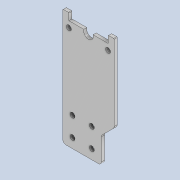
# Autodesk Inventor part: X Axis Statonary Composite Belt Holder RIGHT
Saved by Autodesk Inventor 2022 (Build 260153000, 153)
## iProperties
Created: 2021-10-21
Part Number: X Axis Statonary Composite Belt Holder RIGHT
Material: Generic
Document SubType Name: Modeling
Designer: Coy
Density: 1 g/cm^3
Appearance: Machined - Aluminum
Author: Coy
Autodesk Inventor part; units mm, degrees
ref_plane "YZ Plane" through (0, 0, 0) normal (1, 0, 0) x (0, 1, 0)
ref_plane "XZ Plane" through (0, 0, 0) normal (0, 1, 0) x (-1, 0, 0)
ref_plane "XY Plane" through (0, 0, 0) normal (0, 0, 1) x (1, 0, 0)
sketch "Sketch1" plane through (0, 0, 0) normal (0, 0, 1) x (1, 0, 0)
  line L0 (0, 0) -> (-40, 0)
  line L1 (-40, 0) -> (-40, 40)
  line L2 (-40, 40) -> (0, 40)
  line L3 (0, 40) -> (0, 0)
  line L4 (-30, 30) -> (-10, 30) construction
  line L5 (-10, 30) -> (-10, 10) construction
  line L6 (-10, 10) -> (-30, 10) construction
  line L7 (-30, 10) -> (-30, 30) construction
  line L8 (-30, 30) -> (-40, 30) construction
  line L9 (-10, 10) -> (0, 10) construction
  circle A0 centre (-30, 30) radius 2.6
  circle A1 centre (-10, 30) radius 2.6
  circle A2 centre (-10, 10) radius 2.6
  circle A3 centre (-30, 10) radius 2.6
  line L10 (-40, 40) -> (13, 40)
  line L11 (13, 40) -> (13, 100)
  line L12 (13, 100) -> (-40, 100)
  line L13 (-40, 100) -> (-40, 40)
  line L14 (13, 40) -> (0, 27)
  line L15 (-40, 100) -> (13, 100)
  line L16 (13, 100) -> (13, 120)
  line L17 (-40, 120) -> (-40, 100)
  line L18 (6.75, 120) -> (6.75, 112.72)
  line L19 (6.75, 112.72) -> (-33.75, 112.72)
  line L20 (-33.75, 112.72) -> (-33.75, 120)
  line L21 (-33.75, 112.72) -> (-40, 112.72) construction
  line L22 (6.75, 112.72) -> (13, 112.72) construction
  line L23 (-40, 120) -> (-33.75, 120)
  line L24 (13, 120) -> (6.75, 120)
  line L25 (-13.5, 112.72) -> (-13.5, 111.22) construction
  arc A4 (-18.2697, 112.72) -> (-8.7303, 112.72) centre (-13.5, 111.22) ccw
  dimension "d0" = 40
  dimension "d1" = 40
  dimension "d2" = 5.2
  dimension "d3" = 5.2
  dimension "d4" = 5.2
  dimension "d5" = 5.2
  dimension "d6" = 20
  dimension "d7" = 20
  dimension "d8" = 10
  dimension "d9" = 60
  dimension "d10" = 53
  dimension "d11" = 45
  dimension "d12" = 20
  dimension "d13" = 40.5
  dimension "d14" = 7.28
  dimension "d15" = 1.5
  dimension "d16" = 10
  dimension "d17" = 20
  constraints: 52 end point, 9 perpendicular, 8 parallel, 8 point on line, 6 horizontal, 5 centre point, 5 coincident, 2 equal length, 2 point on circle, 1 collinear, 1 midpoint, 1 vertical
  measures "d0" distance of L0.end L1.end
  measures "d1" distance of L1.end L2.end
  measures "d2" diameter of A0
  measures "d3" diameter of A1
  measures "d4" diameter of A2
  measures "d5" diameter of A3
  measures "d6" distance of L6.end L4.start
  measures "d7" distance of L4.start L4.end
  measures "d8" distance between parallel lines of L0 L6
  measures "d9" distance of L11.end L10.end
  measures "d10" distance of L11.end L12.end
  measures "d11" angle of L10 L14
  measures "d12" distance of L16.end L15.end
  measures "d13" distance of L18.end L19.end
  measures "d14" distance of L18.start L18.end
  measures "d15" distance of L25.start L25.end
  measures "d16" diameter of A4
  measures "d17" distance between parallel lines of L12 L23
extrude "Extrusion1" add sketch "Sketch1" along normal blind 3.175 contours L0 L1 L2 L3 | L3 L10 L14 | L13 L12 L11 L10 L2 | L17 L23 L20 L19 A4 L18 L24 L16 L12
fillet "Fillet1" radius 3.175 4 edges at (0, 0, 1.5875) (-40, 0, 1.5875) (0, 27, 1.5875) (13, 40, 1.5875)
fillet "Fillet2" radius 0.5 4 edges at (13, 120, 1.5875) (-40, 120, 1.5875) (-33.75, 120, 1.5875) (6.75, 120, 1.5875)
sketch "Sketch2" plane through (0, 0, 3.175) normal (0, 0, 1) x (1, 0, 0)
  line L0 (13, 41.3151) -> (13, 119.5) construction
  line L1 (-40, 121.004) -> (13, 121.004) construction
  line L2 (13, 121.004) -> (13, 101.004) construction
  line L3 (13, 101.004) -> (-40, 101.004) construction
  line L4 (-40, 101.004) -> (-40, 121.004) construction
  circle A0 centre (-33.75, 106.36) radius 2.6
  circle A1 centre (6.75, 106.36) radius 2.6
  line L5 (-18.2697, 112.72) -> (-33.75, 112.72) construction
  line L6 (-33.75, 106.36) -> (-33.75, 112.72) construction
  line L7 (6.75, 112.72) -> (-8.7303, 112.72) construction
  line L8 (6.75, 106.36) -> (6.75, 112.72) construction
  point P0 (0, 0)
  dimension "d22" = 20
  dimension "d23" = 5.2
  dimension "d24" = 5.2
  dimension "d25" = 6.36
  dimension "d26" = 6.36
  constraints: 12 end point, 3 perpendicular, 2 centre point, 2 parallel, 1 horizontal, 1 point on line
  measures "d22" distance of L1.end L2.end
  measures "d23" diameter of A0
  measures "d24" diameter of A1
  measures "d25" distance of L6.start L5.end
  measures "d26" distance of L8.start L7.start
extrude "Extrusion2" cut sketch "Sketch2" against normal up to next
equation "\"d3\" = d2"
equation "\"d4\" = d2"
equation "\"d5\" = d2"
equation "\"d24\" = d23"
equation "\"d26\" = d25"
body "Solid1"
